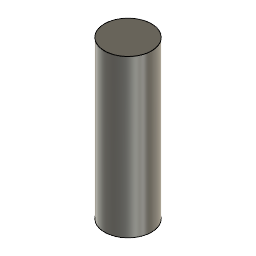
assembly (Autodesk Fusion 360 archive; units mm, degrees)
design "pin"
part number: 2026-06-05-21-15-01-576
Autodesk Fusion 360 part; units mm, degrees
note: some values were not read from the file. Chosen so that the rebuilt part matches the saved one: a direction; which face or edge a step refers to. Set by a fixed rule: which sketch regions a step uses.
sketch "Sketch1" plane through (0, 0, 0) normal (0, 0, 1) x (1, 0, 0)
  circle A0 centre (0, 0) radius 2.4
  dimension "d1" = 4.8
  constraint coincident A0.centre origin
  measures "d1" diameter of A0
extrude "Extrude1" add sketch "Sketch1" along normal blind 16

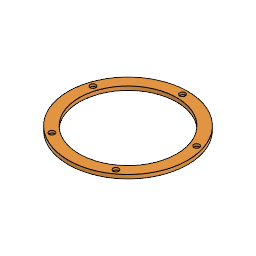
design "Frame-cap"
part number: 2026-05-19-16-44-30-295
Autodesk Fusion 360 part; units mm, degrees
sketch "Sketch1" plane through (0, 0, 0) normal (0, 0, 1) x (1, 0, 0)
  circle A0 centre (0, 0) radius 44
  circle A1 centre (0, 0) radius 54
  line L0 (0, 0) -> (0, 49.2393) construction
  circle A2 centre (0, 49.2393) radius 2.5
  circle A3 centre (-46.8293, 15.2158) radius 2.5
  circle A4 centre (-28.9421, -39.8354) radius 2.5
  circle A5 centre (28.9421, -39.8354) radius 2.5
  circle A6 centre (46.8293, 15.2158) radius 2.5
  dimension "d1" = 88
  dimension "d2" = 108
  dimension "d3" = 49.2393
  dimension "d4" = 5
  dimension "d6" = 360
  constraint coincident A0.centre A1.centre
  constraint concentric A0 A1
  constraint vertical L0
  constraint coincident L0.end A2.centre
  measures "d1" diameter of A0
  measures "d2" diameter of A1
  measures "d3" distance of A0.centre L0.end
  measures "d4" diameter of A2
extrude "Extrude1" add sketch "Sketch1" along normal blind 1.5 contours A2 | A3 | A4 | A5 | A6 makes body 1 at (49.3262, 15.0912, 1) makes body 2 at (2.4969, 49.1147, 1) makes body 3 at (31.439, -39.96, 1) makes body 4 at (-44.3324, 15.0912, 1) makes body 5 at (-26.4452, -39.96, 1)
extrude "Extrude2" add sketch "Sketch1" along normal blind 3.5 bodies 1 2 3 4 5

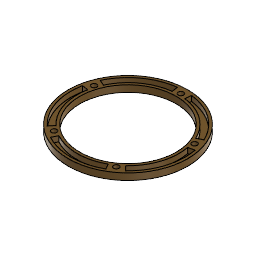
design "Ring"
part number: 2026-05-19-16-03-05-097
Autodesk Fusion 360 part; units mm, degrees
sketch "Sketch1" plane through (0, 0, 0) normal (0, 0, 1) x (1, 0, 0)
  circle A0 centre (0, 0) radius 54.5
  circle A1 centre (0, 0) radius 67.5
  line L0 (0, 0) -> (67.5, 0) construction
  line L1 (0, 0) -> (67.5, 0) construction
  line L2 (0, 56.25) -> (0, 63.25) construction
  circle A2 centre (0, 59.75) radius 3
  line L3 (-7.1543, 57.0532) -> (-8.2283, 63.973)
  line L4 (7.0818, 57.0622) -> (7.7138, 64.0371)
  line L5 (-56.4716, 10.8263) -> (-63.3846, 11.9432)
  circle A3 centre (-56.8256, 18.4638) radius 3
  line L6 (-52.081, 24.3683) -> (-58.5192, 27.1248)
  line L7 (-27.7471, -50.3622) -> (-30.9456, -56.5917)
  circle A4 centre (-35.1202, -48.3388) radius 3
  line L8 (-39.2696, -42.0018) -> (-43.8806, -47.273)
  line L9 (39.323, -41.9518) -> (44.2592, -46.9188)
  circle A5 centre (35.1202, -48.3388) radius 3
  line L10 (27.8111, -50.3269) -> (31.3995, -56.3411)
  line L11 (52.05, 24.4345) -> (58.2993, 27.5943)
  circle A6 centre (56.8256, 18.4638) radius 3
  line L12 (56.4578, 10.8981) -> (63.2866, 12.4523)
  arc A7 (52.05, 24.4345) -> (7.0818, 57.0622) centre (0, 0) ccw
  arc A8 (58.2993, 27.5943) -> (7.7138, 64.0371) centre (0, 0) ccw
  arc A9 (-7.1543, 57.0532) -> (-52.081, 24.3683) centre (0, 0) ccw
  arc A10 (-8.2283, 63.973) -> (-58.5192, 27.1248) centre (0, 0) ccw
  arc A11 (-56.4716, 10.8263) -> (-39.2696, -42.0018) centre (0, 0) ccw
  arc A12 (-63.3846, 11.9432) -> (-43.8806, -47.273) centre (0, 0) ccw
  arc A13 (-27.7471, -50.3622) -> (27.8111, -50.3269) centre (0, 0) ccw
  arc A14 (39.323, -41.9518) -> (56.4578, 10.8981) centre (0, 0) ccw
  arc A15 (-30.9456, -56.5917) -> (31.3995, -56.3411) centre (0, 0) ccw
  arc A16 (44.2592, -46.9188) -> (63.2866, 12.4523) centre (0, 0) ccw
  line L13 (0, 0) -> (0, 67.5) construction
  dimension "d1" = 109
  dimension "d2" = 135
  dimension "d3" = 115
  dimension "d4" = 129
  dimension "d7" = 6
  dimension "d8" = 7
  dimension "d10" = 360
  dimension "d11" = 59.75
  dimension "d12" = 14
  dimension "d14" = 7.2954
  dimension "d15" = 14.8681
  constraint coincident A0.centre A1.centre
  constraint concentric A1 A11
  constraint concentric A11 A12
  constraint horizontal L0
  constraint horizontal L1
  constraint vertical L2
  constraint midpoint L2 A2.centre
  constraint concentric A7 A9
  constraint concentric A8 A10
  constraint concentric A9 A11
  constraint concentric A10 A12
  constraint concentric A11 A13
  constraint concentric A12 A15
  constraint concentric A13 A14
  constraint concentric A15 A16
  constraint coincident L0.end L1.end
  constraint parallel L2 L13
  constraint coincident A2.centre L13
  constraint coincident A1 L13.end
  measures "d1" diameter of A0
  measures "d2" diameter of A1
  measures "d3" diameter of A9
  measures "d4" diameter of A10
  measures "d7" diameter of A2
  measures "d8" distance of L2.start L2.end
  measures "d11" vertical distance of A2.centre A0.centre
  measures "d12" angle of L3 L4
  measures "d14" distance of A2.centre L4
  measures "d15" horizontal distance of L4.end L3.start
extrude "Extrude1" add sketch "Sketch1" along normal blind 1.5 contours A2 | L3 L6 A9 A10 | L4 L11 A7 A8 | L5 L8 A11 A12 | A3 | L7 L10 A13 A15 | A4 | L9 L12 A14 A16 | A5 | A6 makes body 1 at (34.6202, -46.3461, 0) makes body 2 at (61.3877, 8.8614, 0) makes body 3 at (-54.8723, 28.9138, 0) makes body 4 at (-44.4551, -43.2519, 0) makes body 5 at (59.8219, 18.3142, 1) makes body 6 at (-53.8294, 18.3142, 1) makes body 7 at (27.3976, -55.6449, 0) makes body 8 at (10.5421, 61.1215, 0) makes body 9 at (-34.2393, -47.0468, 0) makes body 10 at (2.9963, 59.6005, 1)
extrude "Extrude2" add sketch "Sketch1" along normal blind 7.5 bodies 1 2 3 4 5 6 7 8 9 10

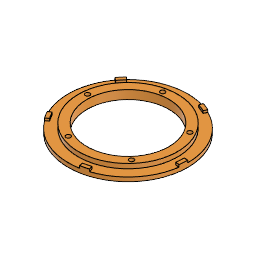
design "Frame-Top"
part number: 2026-05-19-19-00-25-859
Autodesk Fusion 360 part; units mm, degrees
sketch "Sketch1" plane through (0, 0, 0) normal (0, 0, 1) x (1, 0, 0)
  circle A0 centre (0, 0) radius 65
  circle A1 centre (0, 0) radius 44.5
  circle A2 centre (0, 0) radius 54
  line L0 (44.5, 30.59) -> (44.5, 0) construction
  line L1 (-10.3681, 43.2753) -> (-10.3681, 52.9953) construction
  circle A3 centre (-10.3681, 48.1353) radius 2.5
  circle A4 centre (-48.9833, 5.014) radius 2.5
  circle A5 centre (-19.9052, -45.0365) radius 2.5
  circle A6 centre (36.6812, -32.8481) radius 2.5
  circle A7 centre (42.5755, 24.7353) radius 2.5
  line L2 (0, 0) -> (65, 0) construction
  line L3 (0, 0) -> (65, 0) construction
  line L4 (18.85, 58.0144) -> (20.0861, 61.8187)
  line L5 (26.7406, 54.8264) -> (28.4941, 58.4216)
  line L6 (-49.35, 35.8549) -> (-52.5861, 38.206)
  line L7 (-43.8797, 42.3742) -> (-46.7571, 45.1528)
  line L8 (-49.35, -35.8549) -> (-52.5861, -38.206)
  line L9 (-53.8598, -28.6378) -> (-57.3916, -30.5157)
  line L10 (18.85, -58.0144) -> (20.0861, -61.8187)
  line L11 (10.5925, -60.0733) -> (11.2871, -64.0125)
  line L12 (61, 0) -> (65, 0)
  line L13 (60.4064, -8.4896) -> (64.3674, -9.0463)
  arc A8 (26.7406, 54.8264) -> (18.85, 58.0144) centre (0, 0) ccw
  arc A9 (60.4064, -8.4896) -> (61, 0) centre (0, 0) ccw
  arc A10 (-43.8797, 42.3742) -> (-49.35, 35.8549) centre (0, 0) ccw
  arc A11 (-53.8598, -28.6378) -> (-49.35, -35.8549) centre (0, 0) ccw
  arc A12 (10.5925, -60.0733) -> (18.85, -58.0144) centre (0, 0) ccw
  line L14 (0, 0) -> (42.5755, 24.7353) construction
  line L15 (0, 0) -> (0, -65) construction
  dimension "d1" = 130
  dimension "d2" = 89
  dimension "d3" = 108
  dimension "d4" = 5
  dimension "d6" = 360
  dimension "d11" = 360
  dimension "d22" = 30.156
  dimension "d23" = 61
  dimension "d24" = 10
  dimension "d26" = 18
  constraint coincident A0.centre A1.centre
  constraint concentric A1 A2
  constraint coincident A2 L0.start
  constraint coincident A1 L0.end
  constraint vertical L0
  constraint tangent A1 L0
  constraint coincident A2 L1.end
  constraint vertical L1
  constraint coincident A1 L1.start
  constraint midpoint L1 A3.centre
  constraint horizontal L2
  constraint coincident A0 L5.end
  constraint horizontal L3
  constraint coincident A0 L4.end
  constraint concentric A0 A10
  constraint concentric A8 A9
  constraint concentric A9 A12
  constraint concentric A10 A11
  constraint concentric A11 A12
  constraint coincident A7.centre L14.end
  constraint coincident L11 A0.centre
  constraint coincident A0.centre L10
  constraint coincident A0 L15.end
  constraint vertical L15
  measures "d1" diameter of A0
  measures "d2" diameter of A1
  measures "d3" diameter of A2
  measures "d4" diameter of A3
  measures "d22" angle of L2 L14
  measures "d23" radius of A12
  measures "d24" angle of L11 L15
  measures "d26" angle of L10 L15
extrude "Extrude1" add sketch "Sketch1" along normal blind 7 contours A0 L12 L13 A9 | A0 L4 L5 A8 | A0 L10 L11 A12 | A0 L6 L7 A10 | A0 L8 L9 A11 makes body 1 at (64.8749, -4.0311, 4.6667) makes body 2 at (21.9942, 61.1658, 4.6667) makes body 3 at (16.2137, -62.9453, 4.6667) makes body 4 at (-51.9871, 39.0172, 4.6667) makes body 5 at (-53.1725, -37.3857, 4.6667)
extrude "Extrude2" add sketch "Sketch1" along normal blind 4.5 contours A0 L4 L5 L6 L7 L8 L9 L10 L11 L12 L13 A8 A9 A10 A11 A12 bodies 1 2 3 4 5
extrude "Extrude3" add sketch "Sketch1" along normal blind 9.5 contours A2 bodies 1
extrude "Extrude4" add sketch "Sketch1" along normal blind 1.5 contours A3 | A4 | A5 | A6 | A7 bodies 1

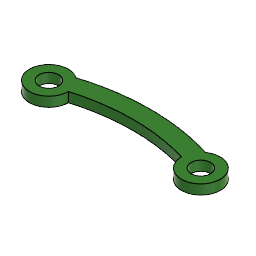
design "Arm"
part number: 2026-05-19-18-27-28-641
Autodesk Fusion 360 part; units mm, degrees
sketch "Sketch1" plane through (0, 0, 0) normal (0, 0, 1) x (1, 0, 0)
  circle A0 centre (39, 0) radius 2.5
  circle A1 centre (0, 0) radius 2.5
  arc A2 (34, 0) -> (5, 0) centre (19.5, -48.8953) ccw
  arc A3 (36.0912, 4.0668) -> (2.9088, 4.0668) centre (19.5, -48.8953) ccw
  arc A4 (2.9088, 4.0668) -> (5, 0) centre (0, 0) ccw
  arc A5 (34, 0) -> (36.0912, 4.0668) centre (39, 0) ccw
  dimension "d1" = 39
  dimension "d2" = 5
  dimension "d3" = 10
  dimension "d4" = 5
  dimension "d5" = 10
  dimension "d6" = 51
  dimension "d7" = 4.5
  dimension "d8" = 34
  constraint concentric A0 A5
  constraint coincident A1.centre A4.centre
  constraint concentric A1 A4
  measures "d1" distance of A1.centre A0.centre
  measures "d2" diameter of A0
  measures "d3" diameter of A5
  measures "d4" diameter of A1
  measures "d5" diameter of A4
  measures "d6" radius of A2
  measures "d8" distance of A1.centre A2.start
extrude "Extrude1" add sketch "Sketch1" along normal blind 2.5

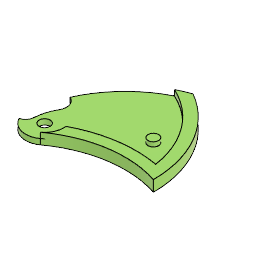
design "Leaf"
part number: 2026-06-05-20-37-06-533
Autodesk Fusion 360 part; units mm, degrees
sketch "Sketch1" plane through (0, 0, 0) normal (0, 0, 1) x (1, 0, 0)
  circle A0 centre (0, 0) radius 49.2 construction
  circle A1 centre (-49.2, 0) radius 2.5
  line L0 (0, 0) -> (-15.2036, -46.792) construction
  line L1 (0, 0) -> (44.5, 0) construction
  circle A2 centre (-49.2, 0) radius 8.6381
  arc A3 (-24.6, 42.6084) -> (-57.7848, 0.9582) centre (-8.0933, -4.5883) ccw
  line L2 (-49.2, 0) -> (0, 0) construction
  arc A4 (0, 0) -> (-24.6, 42.6084) centre (-49.2, 0) ccw
  arc A5 (0, 0) -> (-44.1227, -6.9883) centre (-15.2036, -46.792) ccw
  arc A6 (-5.485, 6.5296) -> (-30.5627, 40.0786) centre (-49.2, 0) ccw
  arc A7 (-5.485, 6.5296) -> (-40.629, 1.0744) centre (-15.2036, -46.792) ccw
  line L3 (0, 0) -> (-16.9706, 16.9706) construction
  circle A8 centre (-16.9706, 16.9706) radius 2.4
  dimension "d1" = 98.4
  dimension "d2" = 5
  dimension "d5" = 50
  dimension "d9" = 72
  dimension "d12" = 4.8
  dimension "d13" = 5
  dimension "d14" = 5
  dimension "d15" = 24
  dimension "d20" = 45
  constraint coincident A0.centre L0.start
  constraint coincident A0 A1.centre
  constraint concentric A1 A4
  constraint horizontal L1
  constraint coincident A0 L0.end
  constraint concentric A1 A2
  constraint coincident A0 A3.start
  constraint coincident A2 A3.end
  constraint tangent A2 A3
  constraint horizontal A0.centre A1.centre
  constraint coincident A1.centre A2.centre
  constraint coincident L0 A0.centre
  constraint coincident A0.centre A5
  constraint tangent A2 A5
  constraint coincident L0.end A5.centre
  constraint coincident A2 A5.end
  constraint coincident A2 A7.end
  constraint coincident A3 A6.end
  constraint coincident L3.end A8.centre
  measures "d1" diameter of A0
  measures "d2" diameter of A1
  measures "d5" radius of A3
  measures "d9" angle of L0 L2
  measures "d12" diameter of A8
  measures "d13" distance of A4 A6
  measures "d14" distance of A5 A7
  measures "d15" distance of A0.centre L3.end
  measures "d20" angle of L2 L3
extrude "Extrude1" add sketch "Sketch1" along normal blind 2.5 contours A2 | A2 A3 A4 A5 A6 A7 | A2 A3 A6 A7 | A8
extrude "Extrude2" add sketch "Sketch1" along normal blind 5 contours A2 A3 A4 A5 A6 A7
extrude "Extrude3" add sketch "Sketch1" along normal blind 4.5 contours A8
sketch "Sketch2" plane through (0, 0, 2.5) normal (0, 0, 1) x (-1, 0, 0)
  circle A0 centre (16.9706, -16.9706) radius 2.4
  arc A1 (44.1227, 6.9883) -> (40.629, -1.0744) centre (49.2, 0) ccw
  arc A2 (5.485, -6.5296) -> (40.629, -1.0744) centre (15.2036, 46.792) ccw
  arc A3 (5.485, -6.5296) -> (30.5627, -40.0786) centre (49.2, 0) ccw
  arc A4 (30.5627, -40.0786) -> (57.7848, -0.9582) centre (8.0933, 4.5883) ccw
  arc A5 (57.7848, -0.9582) -> (44.1227, 6.9883) centre (49.2, 0) ccw
  circle A6 centre (49.2, 0) radius 2.5
  circle A7 centre (57.8824, 0) radius 4
  circle A8 centre (55.5172, -11.2541) radius 5
  arc A9 (51.1977, -8.7358) -> (53.8886, 0.2229) centre (33.9197, 1.3375) ccw
  line L0 (61.8536, -0.4792) -> (60.4812, -11.8531)
  dimension "d21" = 8
  dimension "d22" = 10
  dimension "d23" = 11.5
  dimension "d24" = 20
  constraint coincident A4 A7.centre
  constraint coincident A4 A8.centre
  constraint coincident A7 A9.end
  constraint tangent A7 A9
  constraint coincident A8 A9.start
  constraint tangent A8 A9
  constraint coincident A7 L0.start
  constraint coincident A8 L0.end
  constraint tangent A8 L0
  constraint horizontal A1.centre A7.centre
  constraint tangent A7 L0
  measures "d21" diameter of A7
  measures "d22" diameter of A8
  measures "d23" distance of A7.centre A8.centre
  measures "d24" radius of A9
extrude "Extrude4" cut sketch "Sketch2" against normal through all contours A4 A5 A7 | A4 A5 A7 | A4 A7 A8 A9 | A4 A8 | A4 A8

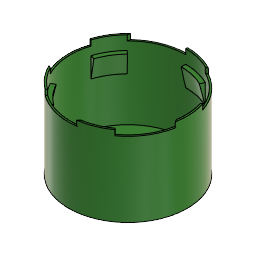
design "frame-base"
part number: 2026-06-05-14-14-42-148
Autodesk Fusion 360 part; units mm, degrees
sketch "Sketch1" plane through (0, 0, 0) normal (0, 0, 1) x (1, 0, 0)
  circle A0 centre (0, 0) radius 65.5
  circle A1 centre (0, 0) radius 67.5
  line L0 (0, 0) -> (0, 65.5)
  line L1 (0, 0) -> (29.226, 58.6182)
  line L2 (29.226, 58.6182) -> (32.4791, 59.1723)
  line L3 (0, 65.5) -> (0, 67.5)
  line L4 (-62.2942, 20.2406) -> (-64.1963, 20.8586)
  line L5 (-46.7179, 45.9096) -> (-46.2396, 49.1747)
  line L6 (-38.4999, -52.9906) -> (-39.6755, -54.6086)
  line L7 (-58.0992, -30.2445) -> (-61.0567, -28.7806)
  line L8 (38.4999, -52.9906) -> (39.6755, -54.6086)
  line L9 (10.8106, -64.6017) -> (8.5044, -66.9621)
  line L10 (62.2942, 20.2406) -> (64.1963, 20.8586)
  line L11 (64.7805, -9.6815) -> (66.3128, -12.6042)
  line L12 (0, 60.5) -> (0, 65.5)
  line L13 (26.995, 54.1435) -> (29.226, 58.6182)
  arc A2 (26.995, 54.1435) -> (0, 60.5) centre (0, 0) ccw
  line L14 (-57.5389, 18.6955) -> (-62.2942, 20.2406)
  arc A3 (-43.1517, 42.405) -> (-57.5389, 18.6955) centre (0, 0) ccw
  line L15 (-43.1517, 42.405) -> (-46.7179, 45.9096)
  line L16 (-35.561, -48.9455) -> (-38.4999, -52.9906)
  arc A4 (-53.6642, -27.9358) -> (-35.561, -48.9455) centre (0, 0) ccw
  line L17 (-53.6642, -27.9358) -> (-58.0992, -30.2445)
  line L18 (35.561, -48.9455) -> (38.4999, -52.9906)
  arc A5 (9.9854, -59.6703) -> (35.561, -48.9455) centre (0, 0) ccw
  line L19 (9.9854, -59.6703) -> (10.8106, -64.6017)
  line L20 (57.5389, 18.6955) -> (62.2942, 20.2406)
  arc A6 (59.8355, -8.9425) -> (57.5389, 18.6955) centre (0, 0) ccw
  line L21 (59.8355, -8.9425) -> (64.7805, -9.6815)
  dimension "d1" = 131
  dimension "d2" = 135
  dimension "d3" = 26.5
  dimension "d4" = 3.3
  dimension "d8" = 360
  dimension "d13" = 121
  dimension "d15" = 360
  constraint coincident A0.centre A1.centre
  constraint concentric A0 A1
  constraint vertical L0
  constraint coincident A0 L1.end
  constraint coincident A0 L0.end
  constraint coincident A1 L2.end
  constraint coincident A1 L3.end
  constraint parallel L0 L3
  constraint concentric A0 A2
  constraint coincident L0 L12.start
  constraint coincident L1 L13.start
  measures "d1" diameter of A0
  measures "d2" diameter of A1
  measures "d3" angle of L0 L1
  measures "d4" distance of L1.end L2.end
  measures "d13" diameter of A2
extrude "Extrude1" add sketch "Sketch1" along normal blind 2.5 contours A0 L20 A6 L21 | A0 L0 L1 L12 L13 L14 A3 L15 L16 A4 L17 L18 A5 L19 L20 A6 L21 | A0 L0 L1 L12 L13 A2 | A0 L18 A5 L19 | L0 L1 A2 | A0 L14 A3 L15 | A0 L16 A4 L17 makes body 1
extrude "Extrude2" add sketch "Sketch1" along normal blind 85 contours A0 A1 L2 L10 | A0 A1 L8 L11 | A0 A1 L3 L5 | A0 A1 L6 L9 | A0 A1 L4 L7 bodies 1
extrude "Extrude3" add sketch "Sketch1" along normal blind 91 contours A0 A1 L10 L11 | A0 A1 L2 L3 | A0 A1 L8 L9 | A0 A1 L4 L5 | A0 A1 L6 L7 bodies 1
extrude "Extrude4" add sketch "Sketch1" along normal blind 23 from surface at 52.5 separate body contours A0 L20 A6 L21 | A0 L0 L1 L12 L13 A2 | A0 L18 A5 L19 | A0 L14 A3 L15 | A0 L16 A4 L17 makes body 2 at (-40.5132, -51.4677, 67.8333) makes body 3 at (-48.4522, 44.0753, 67.8333) makes body 4 at (22.9832, -61.3353, 67.8333) makes body 5 at (2.5239, 65.4514, 67.8333) makes body 6 at (65.3337, -4.6641, 67.8333)
sketch "Sketch2" plane through (0, 0, 0) normal (-0.147809, -0.989016, 0) x (0.989016, -0.147809, 0)
  line L0 (60.5, 52.5) -> (65.5, 52.5)
  line L1 (65.5, 52.5) -> (65.5, 75.5)
  line L2 (65.5, 75.5) -> (60.5, 75.5)
  line L3 (60.5, 75.5) -> (60.5, 52.5)
  line L4 (60.5, 75.5) -> (65.5, 52.5)
  constraint coincident L2.end L3.start
  constraint coincident L0.end L1.start
revolve "Revolve1" cut sketch "Sketch2" angle 360 about axis through (0, 0, 1.75) along (0, 0, 1) contours L0 L3 L4 bodies 2 3 4 5 6
equation "d1 = ( 65.5 * 2 ) * 1 mm"
equation "d2 = ( 67.5 * 2 ) * 1 mm"

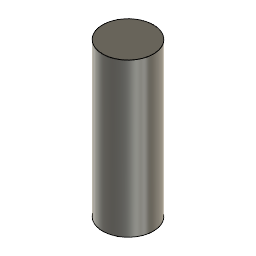
design "pin-ext"
part number: 2026-06-05-22-34-36-345
Autodesk Fusion 360 part; units mm, degrees
sketch "Sketch1" plane through (0, 0, 0) normal (0, 0, 1) x (1, 0, 0)
  circle A0 centre (0, 0) radius 2.4
  dimension "d1" = 4.8
  constraint coincident A0.centre origin
  measures "d1" diameter of A0
extrude "Extrude1" add sketch "Sketch1" along normal blind 14.5
